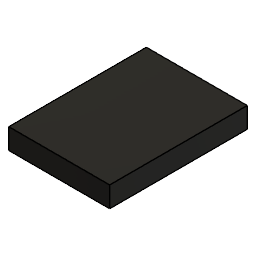
Palitos (Autodesk Fusion 360 design; units mm, degrees)
Autodesk Fusion 360 part; units mm, degrees
sketch "Boceto1" plane through (0, 0, 0) normal (0, 1, 0) x (1, 0, 0)
  line L0 (0, 0) -> (12, 0)
  line L1 (12, 0) -> (17, 0)
  line L2 (17, 0) -> (17, -30)
  line L3 (17, -30) -> (0, -30)
  line L4 (0, -30) -> (-5, -30)
  line L5 (-5, -30) -> (-5, 0)
  line L6 (-5, 0) -> (0, 0)
  line L7 (0, 0) -> (0, -25)
  line L8 (0, -25) -> (12, -25)
  line L9 (12, -25) -> (12, 0)
  dimension "d1" = 12
  dimension "d2" = 5
  dimension "d3" = 30
  dimension "d4" = 5
  constraint coincident L0.start L6.end
  constraint horizontal L0
  constraint parallel L0 L1
  constraint perpendicular L1 L2
  constraint perpendicular L2 L3
  constraint perpendicular L2 L4
  constraint perpendicular L4 L5
  constraint perpendicular L5 L6
  constraint perpendicular L0 L7
  constraint perpendicular L7 L8
  constraint perpendicular L1 L9
  measures "d1" distance of L0.start L0.end
  measures "d2" distance of L0.end L1.end
  measures "d3" distance of L1.end L2.end
  measures "d4" distance of L3.end L4.end
extrude "Extruir1" add sketch "Boceto1" along normal blind 2.5 contours L1 L2 L3 L4 L5 L6 L7 L8 L9
sketch "Boceto2" plane through (0, 2.5, 0) normal (0, 1, 0) x (-1, 0, 0)
  line L0 (-12, 25) -> (0, 25)
  line L1 (0, 25) -> (0, 0)
  line L2 (0, 0) -> (5, 0)
  line L3 (5, 0) -> (5, 30)
  line L4 (5, 30) -> (-17, 30)
  line L5 (-17, 30) -> (-17, 0)
  line L6 (-17, 0) -> (-12, 0)
  line L7 (-12, 0) -> (-12, 25)
  line L8 (5, 0) -> (-17, 0)
  line L9 (-17, 30) -> (-17, 0)
  line L10 (-17, 30) -> (5, 30)
  line L11 (5, 0) -> (5, 30)
  constraint coincident L2.end L3.start
  constraint coincident L5.end L6.start
  constraint coincident L4.end L5.start
  constraint coincident L3.end L4.start
extrude "Extruir2" add sketch "Boceto2" along normal blind 2
